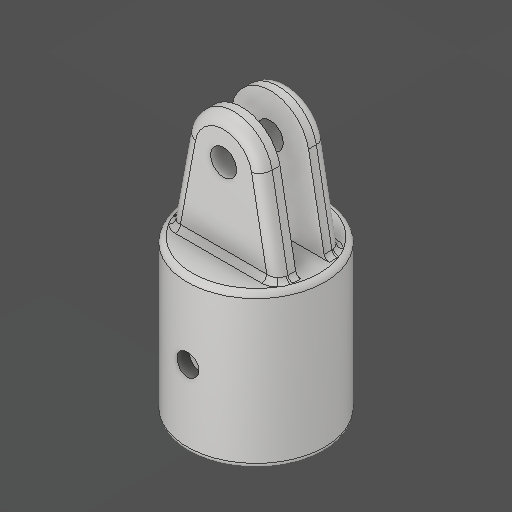
# Autodesk Inventor part: LF50-7
Saved by Autodesk Inventor 2021 (Build 250183000, 183)
## iProperties
Created: 2020-04-23
Part Number: LF50-7
Material: Aluminum 6061 T6 80 Hot Formed
Document SubType Name: Modeling
Designer: Hannah
Density: 2.7 g/cm^3
Appearance: Satin
Author: Hannah
Autodesk Inventor part; units mm, degrees
ref_plane "YZ Plane" through (0, 0, 0) normal (1, 0, 0) x (0, 1, 0)
ref_plane "XZ Plane" through (0, 0, 0) normal (0, 1, 0) x (-1, 0, 0)
ref_plane "XY Plane" through (0, 0, 0) normal (0, 0, 1) x (1, 0, 0)
sketch "Sketch2" plane through (0, 0, 0) normal (0, 1, 0) x (-1, 0, 0)
  circle A0 centre (0, 0) radius 22
  circle A1 centre (0, 0) radius 26.5
  dimension "d5" = 44
  dimension "d6" = 53
  constraints: 2 centre point, 2 coincident
  measures "d5" diameter of A0
  measures "d6" diameter of A1
extrude "Extrusion2" add sketch "Sketch2" along normal mid plane 59 contours A0 | A1
extrude "Extrusion3" cut sketch "Sketch2" along normal blind 24.5 and the other way blind 29.5 contours A0
hole "Hole1" at (0, 0, 0) direction (0, 0, 1) diameter 8.376 end through all thread size "M10x1.5" class "6H" standard "ISO Metric profile"
sketch "Sketch3" plane through (0, 0, 0) normal (0, 0, 1) x (1, 0, 0)
  circle A0 centre (0, 60.5) radius 5
  arc A1 (14.7439, 63.2601) -> (-14.7439, 63.2601) centre (0, 60.5) ccw
  line L0 (-21.064, 29.5) -> (-14.7439, 63.2601)
  line L1 (14.7439, 63.2601) -> (21.064, 29.5)
  line L2 (22, 24.5) -> (-22, 24.5) projected
  line L3 (-26.5, -29.5) -> (26.5, -29.5) projected
  line L4 (26.5, 29.5) -> (-26.5, 29.5) projected
  line L5 (-21.064, 29.5) -> (21.064, 29.5)
  point P0 (0, 0)
  dimension "d36" = 10
  dimension "d37" = 15
  dimension "d50" = 90
  constraints: 6 end point, 4 point on line, 2 centre point, 2 point on circle, 2 tangent, 1 coincident, 1 equal length
  measures "d36" diameter of A0
  measures "d37" radius of A1
  measures "d50" distance from line of L3 A0.centre
extrude "Extrusion5" add sketch "Sketch3" along normal mid plane 25
extrude "Extrusion6" cut sketch "Sketch3" along normal mid plane 11
fillet "Fillet2" radius 4 6 edges at (0, 75.5, 12.5) (17.9039, 46.3801, 12.5) (-17.9039, 46.3801, 12.5) (0, 75.5, -12.5) (17.9039, 46.3801, -12.5) (-17.9039, 46.3801, -12.5)
fillet "Fillet2" radius 2 2 edges at (26.5, 29.5, 0) (26.5, -29.5, 0)
fillet "Fillet3" radius 2 10 edges at (-19.872, 29.5, 11.3284) (-21.064, 29.5, 7) (19.872, 29.5, 11.3284) (21.064, 29.5, 7) (0, 29.5, 12.5) (19.872, 29.5, -11.3284) (0, 29.5, -12.5) (-19.872, 29.5, -11.3284) (-21.064, 29.5, -7) (21.064, 29.5, -7)
equation "\"d46\" = 0.5 * d7"
equation "\"d7\" = 59"
body "Solid1"
